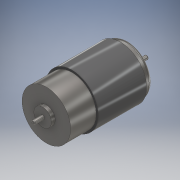
# Autodesk Inventor part: JD5B-2655W-R
Saved by Autodesk Inventor 2018 (Build 220112000, 112)
## iProperties
Created: 2018-01-11
Part Number: JD5B-2655W-R
Material: Generic
Document SubType Name: Modeling
Designer: Moochster
Density: 1 g/cm^3
Appearance: Semi-Polished
Author: Moochster
Autodesk Inventor part; units mm, degrees
ref_plane "YZ Plane" through (0, 0, 0) normal (1, 0, 0) x (0, 1, 0)
ref_plane "XZ Plane" through (0, 0, 0) normal (0, 1, 0) x (-1, 0, 0)
ref_plane "XY Plane" through (0, 0, 0) normal (0, 0, 1) x (1, 0, 0)
sketch "Sketch1" plane through (0, 0, 0) normal (0, 0, 1) x (1, 0, 0)
  line L0 (0, 0) -> (0, 64.76)
  line L1 (0, 0) -> (1.115, 0)
  line L2 (1.115, 0) -> (1.115, 5.6)
  line L3 (1.115, 5.6) -> (5, 5.6)
  line L4 (5, 5.6) -> (5, 7.7)
  line L5 (5, 7.7) -> (13.77, 7.7)
  line L6 (13.77, 7.7) -> (13.77, 54.2)
  line L7 (13.77, 54.2) -> (5, 54.2)
  line L8 (5, 54.2) -> (5, 56.56)
  line L9 (5, 56.56) -> (1.115, 56.56)
  line L10 (1.115, 56.56) -> (1.115, 64.76)
  line L11 (1.115, 64.76) -> (0, 64.76)
  line L12 (13.77, 49.7) -> (14.865, 49.7)
  line L13 (14.865, 49.7) -> (14.865, 22.2)
  line L14 (14.865, 22.2) -> (13.77, 22.2)
  dimension "d0" = 2.23
  dimension "d1" = 5.6
  dimension "d2" = 8.2
  dimension "d3" = 2.36
  dimension "d4" = 2.1
  dimension "d5" = 10
  dimension "d6" = 10
  dimension "d7" = 46.5
  dimension "d8" = 27.54
  dimension "d9" = 14.5
  dimension "d10" = 27.5
  dimension "d11" = 29.73
  constraints: 30 end point, 11 perpendicular, 3 horizontal, 2 point on line, 1 vertical, 1 vertical alignment
  measures "d0" diameter of L2 L0
  measures "d1" distance of L1.end L2.end
  measures "d2" distance of L9.end L10.end
  measures "d3" distance of L7.end L8.end
  measures "d4" distance of L3.end L4.end
  measures "d5" diameter of L8 L0
  measures "d6" diameter of L4 L0
  measures "d7" distance of L5.end L6.end
  measures "d8" diameter of L6 L0
  measures "d9" distance from line of L5.end L14
  measures "d10" distance of L12.end L13.end
  measures "d11" diameter of L13 L0
revolve "Revolution1" add sketch "Sketch1" angle 360 about axis through (0, 0, 0) along (0, 1, 0) contours L0 L11 L10 L9 L8 L7 L6 L5 L4 L3 L2 L1
revolve "Revolution2" add sketch "Sketch1" angle 345 mid plane about axis through (0, 0, 0) along (0, 1, 0) contours L6 L12 L13 L14
fillet "Fillet1" radius 2 1 edges at (-13.77, 54.2, 0)
fillet "Fillet2" radius 0.5 2 edges at (-1.115, 0, 0) (-1.115, 64.76, 0)
sketch "Sketch2" plane through (0, 54.2, 0) normal (0, 1, 0) x (1, 0, 0)
  point P0 (0, 0)
  point P1 (-10.5, 0)
  point P2 (0, 8)
  point P3 (0, -8)
  dimension "d16" = 10.5
  dimension "d17" = 8
  dimension "d18" = 8
  constraints: 2 vertical alignment, 1 horizontal alignment
  measures "d16" distance of point (-10.5, 0) point (0, 0)
  measures "d17" distance of point (0, 0) point (0, 8)
  measures "d18" distance of point (0, -8) point (0, 0)
hole "Hole1" at (0, 54.2, -8) at (0, 54.2, 8) direction (0, -1, 0) diameter 2 depth 8 tip angle 118
body "Solid1"
